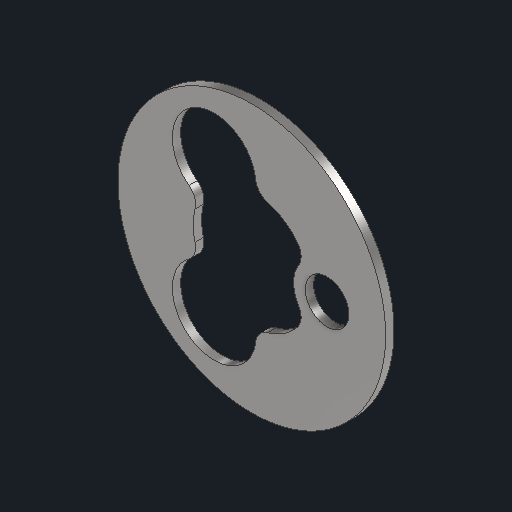
# Autodesk Inventor part: ring-pre-anode
Saved by Autodesk Inventor 2025 (Build 290162000, 162)
## iProperties
Created: 2024-05-14
Part Number: ring-pre-anode
Material: Stainless Steel
Document SubType Name: Modeling
Designer: kuzmin
Density: 8 g/cm^3
Appearance: Semi-Polished
Author: kuzmin
Autodesk Inventor part; units mm, degrees
ref_plane "YZ Plane" through (0, 0, 0) normal (1, 0, 0) x (0, 1, 0)
ref_plane "XZ Plane" through (0, 0, 0) normal (0, 1, 0) x (-1, 0, 0)
ref_plane "XY Plane" through (0, 0, 0) normal (0, 0, 1) x (1, 0, 0)
sketch "Sketch1" plane through (0, 0, 0) normal (0, 0, 1) x (1, 0, 0)
  circle A0 centre (0, 0) radius 7
  circle A1 centre (0, 0) radius 16
  dimension "d0" = 32
  dimension "d1" = 14
  constraints: 2 centre point, 2 coincident
  measures "d0" diameter of A1
  measures "d1" diameter of A0
extrude "Extrusion1" add sketch "Sketch1" along normal blind 1
sketch "Sketch2" plane through (0, 0, 1) normal (0, 0, 1) x (1, 0, 0)
  circle A0 centre (9, 0) radius 2.6
  point P0 (0, 0)
  dimension "d4" = 9
  dimension "d5" = 5.2
  constraints: 1 centre point, 1 horizontal alignment
  measures "d4" distance of point (0, 0) A0.centre
  measures "d5" diameter of A0
extrude "Extrusion2" cut sketch "Sketch2" against normal blind 1
pattern_circular "Circular Pattern1" count 3 over 360 about axis through (0, 0, 0) along (0, 0, 1) of "Extrusion2"
sketch "Sketch4" plane through (0, 0, 1) normal (0, 0, 1) x (1, 0, 0)
  arc A0 (-2.1614, 6.6579) -> (-4.6852, 5.2008) centre (-4.5, 7.7942) ccw projected
  circle A1 centre (-4.5, 7.7942) radius 5
  arc A2 (-4.6852, -5.2008) -> (-2.1614, -6.6579) centre (-4.5, -7.7942) ccw projected
  circle A3 centre (-4.5, -7.7942) radius 5
  point P0 (0, 0)
  dimension "d12" = 10
  constraints: 2 centre point, 2 coincident, 1 equal radius
  measures "d12" diameter of A1
extrude "Extrusion3" cut sketch "Sketch4" against normal through all
sketch "Sketch5" plane through (0, 0, 1) normal (0, 0, 1) x (1, 0, 0)
  arc A0 (6.8467, -1.4571) -> (6.8467, 1.4571) centre (9, 0) ccw projected
  circle A1 centre (9, 0) radius 4
  circle A2 centre (9, 0) radius 2.6
  point P0 (0, 0)
  point P1 (6.8467, 1.4571)
  dimension "d16" = 8
  constraints: 2 centre point, 2 coincident, 1 concentric
  measures "d16" diameter of A1
extrude "Extrusion4" add sketch "Sketch5" against normal up to surface (1 mm away)
fillet "Fillet3" radius 2 6 edges at (0.4343, 6.9865, 0.5) (-6.2677, 3.1171, 0.5) (-6.2677, -3.1171, 0.5) (0.4343, -6.9865, 0.5) (6.3333, -2.9814, 0.5) (6.3333, 2.9814, 0.5)
body "Solid1"
